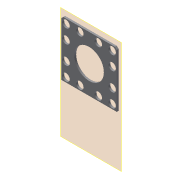
# Autodesk Inventor part: cellSTORM_UC2_motorized_xystage_spacer
Saved by Autodesk Inventor 2019.4 (Build 234330000, 330)
## iProperties
Created: 2021-03-02
Part Number: cellSTORM_UC2_motorized_xystage_spacer
Material: Generic
Document SubType Name: Modeling
Designer: diederichbenedict
Density: 1 g/cm^3
Appearance: Default
Author: diederichbenedict
Autodesk Inventor part; units mm, degrees
ref_plane "YZ Plane" through (0, 0, 0) normal (1, 0, 0) x (0, 1, 0)
ref_plane "XZ Plane" through (0, 0, 0) normal (0, 1, 0) x (-1, 0, 0)
ref_plane "XY Plane" through (0, 0, 0) normal (0, 0, 1) x (1, 0, 0)
ref_plane "Work Plane1" through (0, 0, 0) normal (0, 0, 1) x (1, 0, 0)
sketch "Sketch1" plane through (0, 0, 0) normal (0, 0, 1) x (1, 0, 0)
  circle A0 centre (24.1273, 54.4044) radius 16 projected
  circle A1 centre (34.1273, 29.4044) radius 4 projected
  circle A2 centre (49.1273, 64.4044) radius 4 projected
  circle A3 centre (14.1273, 79.4044) radius 4 projected
  circle A4 centre (-0.8727, 44.4044) radius 4 projected
  circle A5 centre (-0.8727, 64.4044) radius 4 projected
  circle A6 centre (34.1273, 79.4044) radius 4 projected
  circle A7 centre (49.1273, 44.4044) radius 4 projected
  circle A8 centre (14.1273, 29.4044) radius 4 projected
  arc A9 (-5.8727, -21.5956) -> (-1.8727, -25.5956) centre (-1.8727, -21.5956) ccw projected
  line L0 (-1.8727, -25.5956) -> (2.1273, -25.5956) projected
  arc A10 (2.1273, -25.5956) -> (6.1273, -21.5956) centre (2.1273, -21.5956) ccw projected
  line L1 (6.1273, -21.5956) -> (6.1273, 20.4044) projected
  arc A11 (10.1273, 24.4044) -> (6.1273, 20.4044) centre (10.1273, 20.4044) ccw projected
  line L2 (10.1273, 24.4044) -> (38.1273, 24.4044) projected
  arc A12 (42.1273, 20.4044) -> (38.1273, 24.4044) centre (38.1273, 20.4044) ccw projected
  line L3 (42.1273, 20.4044) -> (42.1273, -21.5956) projected
  arc A13 (42.1273, -21.5956) -> (46.1273, -25.5956) centre (46.1273, -21.5956) ccw projected
  line L4 (46.1273, -25.5956) -> (50.1273, -25.5956) projected
  arc A14 (50.1273, -25.5956) -> (54.1273, -21.5956) centre (50.1273, -21.5956) ccw projected
  line L5 (54.1273, -21.5956) -> (54.1273, 82.4044) projected
  line L6 (54.1273, 82.4044) -> (52.1273, 84.4044) projected
  line L7 (52.1273, 84.4044) -> (-3.8727, 84.4044) projected
  line L8 (-3.8727, 84.4044) -> (-5.8727, 82.4044) projected
  line L9 (-5.8727, 82.4044) -> (-5.8727, -21.5956) projected
  line L10 (-5.8727, 84.4044) -> (54.1273, 84.4044)
  line L11 (54.1273, 84.4044) -> (54.1273, 24.4044)
  line L12 (54.1273, 24.4044) -> (-5.8727, 24.4044)
  line L13 (-5.8727, 24.4044) -> (-5.8727, 84.4044)
  line L14 (-5.8727, 84.4044) -> (54.1273, 24.4044) construction
  line L15 (54.1273, 84.4044) -> (-5.8727, 24.4044) construction
  circle A15 centre (24.1273, 54.4044) radius 16 projected
  circle A16 centre (34.1273, 29.4044) radius 4 projected
  circle A17 centre (49.1273, 64.4044) radius 4 projected
  circle A18 centre (14.1273, 79.4044) radius 4 projected
  circle A19 centre (-0.8727, 44.4044) radius 4 projected
  circle A20 centre (-0.8727, 64.4044) radius 4 projected
  circle A21 centre (34.1273, 79.4044) radius 4 projected
  circle A22 centre (49.1273, 44.4044) radius 4 projected
  circle A23 centre (14.1273, 29.4044) radius 4 projected
  arc A24 (-5.8727, -21.5956) -> (-1.8727, -25.5956) centre (-1.8727, -21.5956) ccw projected
  line L16 (-1.8727, -25.5956) -> (2.1273, -25.5956) projected
  arc A25 (2.1273, -25.5956) -> (6.1273, -21.5956) centre (2.1273, -21.5956) ccw projected
  line L17 (6.1273, -21.5956) -> (6.1273, 20.4044) projected
  arc A26 (10.1273, 24.4044) -> (6.1273, 20.4044) centre (10.1273, 20.4044) ccw projected
  line L18 (10.1273, 24.4044) -> (38.1273, 24.4044) projected
  arc A27 (42.1273, 20.4044) -> (38.1273, 24.4044) centre (38.1273, 20.4044) ccw projected
  line L19 (42.1273, 20.4044) -> (42.1273, -21.5956) projected
  arc A28 (42.1273, -21.5956) -> (46.1273, -25.5956) centre (46.1273, -21.5956) ccw projected
  line L20 (46.1273, -25.5956) -> (50.1273, -25.5956) projected
  arc A29 (50.1273, -25.5956) -> (54.1273, -21.5956) centre (50.1273, -21.5956) ccw projected
  line L21 (54.1273, -21.5956) -> (54.1273, 82.4044) projected
  line L22 (54.1273, 82.4044) -> (52.1273, 84.4044) projected
  line L23 (52.1273, 84.4044) -> (-3.8727, 84.4044) projected
  line L24 (-3.8727, 84.4044) -> (-5.8727, 82.4044) projected
  line L25 (-5.8727, 82.4044) -> (-5.8727, -21.5956) projected
  circle A30 centre (49.1273, 29.4044) radius 4 projected
  circle A31 centre (-0.8727, 79.4044) radius 4 projected
  circle A32 centre (-0.8727, 29.4044) radius 4 projected
  circle A33 centre (41.6273, 36.9044) radius 1.95 projected
  circle A34 centre (41.6273, 71.9044) radius 1.95 projected
  circle A35 centre (6.6273, 71.9044) radius 1.95 projected
  circle A36 centre (49.1273, 29.4044) radius 4 projected
  circle A37 centre (-0.8727, 79.4044) radius 4 projected
  circle A38 centre (-0.8727, 29.4044) radius 4 projected
  circle A39 centre (41.6273, 36.9044) radius 1.95 projected
  circle A40 centre (41.6273, 71.9044) radius 1.95 projected
  circle A41 centre (6.6273, 71.9044) radius 1.95 projected
  circle A42 centre (49.1273, 79.4044) radius 4 projected
  circle A43 centre (49.1273, 79.4044) radius 4 projected
  point P0 (0, 0)
  constraints: 12 end point, 2 midpoint, 2 parallel, 1 horizontal, 1 perpendicular, 1 point on line
extrude "Extrusion1" add sketch "Sketch1" along normal blind 2 contours L9 L8 L7 L6 L5 L12 L2 | A33 | A34 | A35
body "Solid1"
